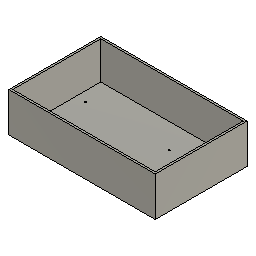
Caja (Autodesk Fusion 360 design; units mm, degrees)
Autodesk Fusion 360 part; units mm, degrees
sketch "Sketch1" plane through (0, 0, 0) normal (0, 0, 1) x (1, 0, 0)
  line L0 (0, 0) -> (223, 0)
  line L1 (223, 0) -> (223, 140)
  line L2 (223, 140) -> (0, 140)
  line L3 (0, 140) -> (0, 0)
  dimension "d1" = 223
  dimension "d2" = 140
  constraint horizontal L0
  constraint vertical L1
  constraint horizontal L2
  constraint vertical L3
  constraint coincident L0.start L3.end
  measures "d1" distance of L0.start L0.end
  measures "d2" distance of L0.end L1.end
extrude "Extrude1" add sketch "Sketch1" along normal blind 60
sketch "Sketch2" plane through (0, 0, 60) normal (0, 0, 1) x (-1, 0, 0)
  line L0 (0, -140) -> (0, 0)
  line L1 (0, 0) -> (-223, 0)
  line L2 (-223, 0) -> (-223, -140)
  line L3 (-223, -140) -> (0, -140)
  line L4 (-3, -137) -> (-220, -137)
  line L5 (-220, -137) -> (-220, -3)
  line L6 (-220, -3) -> (-3, -3)
  line L7 (-3, -3) -> (-3, -137)
  dimension "d5" = 3
  dimension "d6" = 3
  dimension "d7" = 3
  dimension "d8" = 3
  constraint horizontal L4
  constraint vertical L5
  constraint horizontal L6
  constraint vertical L7
  measures "d5" distance of L0 L7
  measures "d6" distance of L1 L6
  measures "d7" distance of L3 L4
  measures "d8" distance of L2 L5
extrude "Extrude2" cut sketch "Sketch2" against normal blind 57 contours L4 L5 L6 L7
sketch "Sketch3" plane through (0, 0, 0) normal (0, 0, -1) x (1, 0, 0)
  line L0 (0, 0) -> (0, -140)
  line L1 (0, -140) -> (223, -140)
  line L2 (223, -140) -> (223, 0)
  line L3 (223, 0) -> (0, 0)
  line L4 (205.0199, -4.8072) -> (6.0134, -4.8072) construction
  line L5 (6.0134, -113.804) -> (205.0199, -113.804) construction
  line L6 (205.0199, -113.804) -> (9.7448, -113.804) construction
  line L7 (205.0199, -59.3055) -> (147.0519, -59.3055) construction
  circle A0 centre (145.0199, -99.104) radius 1.25
  circle A1 centre (145.0199, -19.507) radius 1.25
  circle A2 centre (18.0134, -99.104) radius 1.25
  line L8 (6.0134, -4.8072) -> (6.0134, -113.804) construction
  line L9 (205.0199, -113.804) -> (205.0199, -4.8072) construction
  line L10 (6.0134, -111.0749) -> (6.0134, -6.1412) construction
  circle A3 centre (18.0134, -19.507) radius 1.25
  point P0 (180.3238, -104.2905)
  dimension "d11" = 12
  dimension "d12" = 14.7
  dimension "d13" = 2.5
  dimension "d17" = 108.9968
  dimension "d18" = 54.4985
  dimension "d19" = 2.5
  dimension "d20" = 60
  dimension "d21" = 14.7
  constraint coincident L5.end L6.start
  constraint coincident L7.start L9
  constraint perpendicular L7 L9
  constraint symmetric L7 A2 A3
  constraint symmetric L7 A0 A1
  measures "d11" distance of A2.centre L10
  measures "d12" distance of A2.centre L6
  measures "d13" diameter of A2
  measures "d17" distance of L4 L5
  measures "d18" distance of L5 L7
  measures "d19" diameter of A0
  measures "d20" distance of A0.centre L9
  measures "d21" distance of A0.centre L5
extrude "Extrude3" cut sketch "Sketch3" against normal up to surface (3 mm away) contours A0 | A1 | A2 | A3
